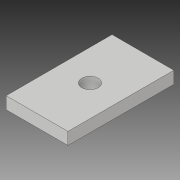
# Autodesk Inventor part: stage_shim
Saved by Autodesk Inventor 2019 (Build 230136000, 136)
## iProperties
Created: 2020-03-09
Part Number: stage_shim
Material: Generic
Document SubType Name: Modeling
Designer: devon
Density: 1 g/cm^3
Appearance: Default
Author: devon
Autodesk Inventor part; units mm, degrees
ref_plane "YZ Plane" through (0, 0, 0) normal (1, 0, 0) x (0, 1, 0)
ref_plane "XZ Plane" through (0, 0, 0) normal (0, 1, 0) x (-1, 0, 0)
ref_plane "XY Plane" through (0, 0, 0) normal (0, 0, 1) x (1, 0, 0)
sketch "Sketch1" plane through (0, 0, 0) normal (0, 1, 0) x (-1, 0, 0)
  line L0 (12.7, 21.75) -> (-12.7, 21.75)
  line L1 (-12.7, 21.75) -> (-12.7, -21.75)
  line L2 (-12.7, -21.75) -> (12.7, -21.75)
  line L3 (12.7, -21.75) -> (12.7, 21.75)
  line L4 (12.7, 21.75) -> (-12.7, -21.75) construction
  line L5 (-12.7, 21.75) -> (12.7, -21.75) construction
  point P0 (0, 0)
  dimension "d0" = 25.4
  dimension "d1" = 43.5
  constraints: 12 end point, 2 midpoint, 2 parallel, 1 horizontal, 1 perpendicular
  measures "d0" distance of L1.end L2.end
  measures "d1" distance of L2.end L0.start
extrude "Extrusion1" add sketch "Sketch1" along normal blind 5
sketch "Sketch2" plane through (0, 5, 0) normal (0, 1, 0) x (1, 0, 0)
  point P0 (0, 0)
  point P1 (0, 0)
  dimension "d11" = 0
  dimension "d12" = 0
  measures "d11" distance of point (0, 0) point (0, 0)
  measures "d12" distance of point (0, 0) point (0, 0)
hole "Hole1" at (0, 5, 0) direction (0, -1, 0) diameter 6.756 depth 25.4 clearance for "Flat Head Machine Screw (82)" size "1/4" standard "Ansi Unified Screw Threads"
body "Solid1"
